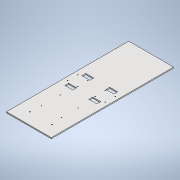
# Autodesk Inventor part: bottom
Saved by Autodesk Inventor 2020 (Build 240168000, 168)
## iProperties
Created: 2021-10-02
Part Number: bottom
Material: Типовые
Document SubType Name: Modeling
Designer: Петров Иван
Density: 1 g/cm^3
Appearance: По умолчанию
Author: Петров Иван
Autodesk Inventor part; units mm, degrees
ref_plane "YZ Plane" through (0, 0, 0) normal (1, 0, 0) x (0, 1, 0)
ref_plane "XZ Plane" through (0, 0, 0) normal (0, 1, 0) x (-1, 0, 0)
ref_plane "XY Plane" through (0, 0, 0) normal (0, 0, 1) x (1, 0, 0)
sketch "Эскиз1" plane through (0, 0, 0) normal (0, 1, 0) x (-1, 0, 0)
  line L0 (-82.5, 225) -> (82.5, 225)
  line L1 (82.5, 225) -> (82.5, -225)
  line L2 (82.5, -225) -> (-82.5, -225)
  line L3 (-82.5, -225) -> (-82.5, 225)
  line L4 (-82.5, 225) -> (82.5, -225) construction
  line L5 (82.5, 225) -> (-82.5, -225) construction
  point P0 (0, 0)
  dimension "d0" = 165
  dimension "d1" = 450
  constraints: 12 end point, 2 midpoint, 2 parallel, 1 horizontal, 1 perpendicular
  measures "d0" distance of L1.end L2.end
  measures "d1" distance of L0.end L1.end
extrude "Выдавливание1" add sketch "Эскиз1" along normal blind 4
sketch "Эскиз3" plane through (0, 0, 0) normal (0, -1, 0) x (1, 0, 0)
  circle A0 centre (42.3945, 182) radius 2 projected
  circle A1 centre (-39.5136, 182) radius 2 projected
  point P0 (0, 0)
extrude "Выдавливание3" cut sketch "Эскиз3" against normal blind 4
sketch "Эскиз4" plane through (0, 4, 0) normal (0, 1, 0) x (1, 0, 0)
  circle A0 centre (37.93, -81.5) radius 1.2889 projected
  circle A1 centre (-37.0605, -72.5) radius 1.2889 projected
  circle A2 centre (-37.0605, -141.5) radius 1.2889 projected
  circle A3 centre (36.93, -141.5) radius 1.2889 projected
  circle A4 centre (32.125, -13) radius 1.5 projected
  circle A5 centre (69.125, -13) radius 1.5 projected
  circle A6 centre (69.125, 24) radius 1.5 projected
  circle A7 centre (32.125, 24) radius 1.5 projected
  circle A8 centre (-32.125, 24) radius 1.5 projected
  circle A9 centre (-69.125, 24) radius 1.5 projected
  circle A10 centre (-69.125, -13) radius 1.5 projected
  circle A11 centre (-32.125, -13) radius 1.5 projected
  point P0 (0, 0)
extrude "Выдавливание4" cut sketch "Эскиз4" against normal blind 4
sketch "Эскиз5" plane through (0, 4, 0) normal (0, 1, 0) x (1, 0, 0)
  line L0 (-58.9065, 28.8404) -> (-29.5747, 28.8404)
  line L1 (-29.5747, 28.8404) -> (-29.5747, 43.2578)
  line L2 (-29.5747, 43.2578) -> (-58.9065, 43.2578)
  line L3 (-58.9065, 43.2578) -> (-58.9065, 28.8404)
  line L4 (-58.9065, 28.8404) -> (-29.5747, 43.2578) construction
  line L5 (-29.5747, 28.8404) -> (-58.9065, 43.2578) construction
  line L6 (-58.9065, -33.8129) -> (-29.5747, -33.8129)
  line L7 (-29.5747, -33.8129) -> (-29.5747, -19.3955)
  line L8 (-29.5747, -19.3955) -> (-58.9065, -19.3955)
  line L9 (-58.9065, -19.3955) -> (-58.9065, -33.8129)
  line L10 (-58.9065, -33.8129) -> (-29.5747, -19.3955) construction
  line L11 (-29.5747, -33.8129) -> (-58.9065, -19.3955) construction
  point P0 (0, 0)
  point P1 (-44.2406, 36.0491)
  point P2 (-44.2406, -26.6042)
  constraints: 24 end point, 4 midpoint, 4 parallel, 2 horizontal, 2 perpendicular
extrude "Выдавливание5" cut sketch "Эскиз5" against normal blind 4
mirror "Зеркальное отражение1" about plane through (0, 0, 0) normal (1, 0, 0) of "Выдавливание5"
